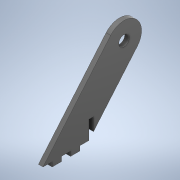
# Autodesk Inventor part: WeaponStandoffBearingV1
Saved by Autodesk Inventor 2020 (Build 240168000, 168)
## iProperties
Created: 2023-11-28
Part Number: WeaponStandoffBearingV1
Material: Thermoplastic Resin
Document SubType Name: Modeling
Designer: smz3rm
Density: 1.28 g/cm^3
Appearance: Smooth - Black
Mass: 5.9667 g
Surface Area: 37.6103 cm^2
Volume: 4.66148 cm^3
Author: smz3rm
Autodesk Inventor part; units mm, degrees
ref_plane "YZ Plane" through (0, 0, 0) normal (1, 0, 0) x (0, 1, 0)
ref_plane "XZ Plane" through (0, 0, 0) normal (0, 1, 0) x (-1, 0, 0)
ref_plane "XY Plane" through (0, 0, 0) normal (0, 0, 1) x (1, 0, 0)
sketch "Sketch1" plane through (0, 0, 0) normal (1, 0, 0) x (0, 1, 0)
  line L0 (0, 0) -> (0, 30)
  line L1 (0, 24) -> (-3, 24)
  line L2 (-3, 24) -> (-3, 18)
  line L3 (-3, 18) -> (0, 18)
  line L4 (0, 6) -> (-3, 6)
  line L5 (-3, 6) -> (-3, 12)
  line L6 (-3, 12) -> (0, 12)
  line L7 (0, 30) -> (52.3941, -14.2439)
  line L8 (0, 0) -> (37.6059, -31.7561)
  circle A0 centre (45, -23) radius 11.4604
  line L9 (0, 0) -> (0, -3)
  line L10 (0, -3) -> (12, -3)
  line L11 (12, -3) -> (12, 0)
  line L12 (12, 0) -> (0, 0)
  point P0 (3.5526, -3)
  dimension "d0" = 30
  dimension "d1" = 3
  dimension "d2" = 6
  dimension "d3" = 3
  dimension "d4" = 6
  dimension "d7" = 6
  dimension "d8" = 6
  dimension "d9" = 45
  dimension "d10" = 23
  dimension "d16" = 3
  dimension "WeaponMountSlot" = 12
  constraints: 26 end point, 4 perpendicular, 4 point on line, 3 parallel, 3 vertical, 2 horizontal, 2 point on circle, 2 tangent, 1 centre point
  measures "d0" distance of L0.start L0.end
  measures "d1" distance of L1.start L1.end
  measures "d2" distance of L1.end L2.end
  measures "d3" distance of L4.start L4.end
  measures "d4" distance of L4.end L5.end
  measures "d7" distance from line of L0.end L1
  measures "d8" distance from line of L0.start L4
  measures "d9" distance from line of L0 A0.centre
  measures "d10" vertical distance of L0.start A0.centre
  measures "d16" distance of L0.start L9.end
  measures "WeaponMountSlot" distance of L9.end L10.end
extrude "Extrusion1" add sketch "Sketch1" along normal blind 3 contours L0 L7 A0 L8 L10 L11 L12 | L4 L5 L6 L0 | A0 | L3 L2 L1 L0
sketch "Sketch3" plane through (3, 0, 0) normal (1, 0, 0) x (0, 0, -1)
  arc A0 (31.7561, 37.6059) -> (14.2439, 52.3941) centre (23, 45) ccw projected
  circle A1 centre (23, 45) radius 3.5
  point P0 (0, 0)
  dimension "d13" = 7
  constraints: 1 centre point, 1 coincident
  measures "d13" diameter of A1
extrude "Extrusion2" cut sketch "Sketch3" against normal up to surface (3 mm away)
equation "\"d1\" = BaseWallThickness"
equation "\"d2\" = TabSize"
equation "\"d3\" = d5"
equation "\"d4\" = d6"
equation "\"d7\" = TabSize"
equation "\"d8\" = TabSize"
equation "\"d9\" = BladeHeight"
equation "\"d10\" = BladeForwardness + SideWallThickness"
equation "\"d16\" = SideWallThickness"
equation "\"d11\" = SideWallThickness"
equation "\"BaseWallThickness\" = 3"
equation "\"SideWallThickness\" = 3"
equation "\"BladeHeight\" = 45"
equation "\"BladeForwardness\" = 20"
equation "\"TabSize\" = 6"
equation "\"d5\" = 3"
equation "\"d6\" = 6"
body "Solid1"
